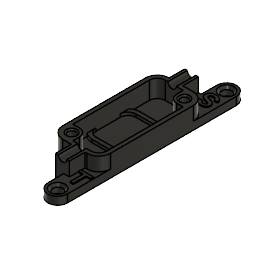
PE3 - PCB Case (Autodesk Fusion 360 design; units mm, degrees)
Autodesk Fusion 360 part; units mm, degrees
sketch "Sketch1" plane through (0, 0, 0) normal (0, 0, 1) x (1, 0, 0)
  line L0 (6.2013, 10.25) -> (-6.2012, 10.25)
  line L1 (-10.25, 6.2013) -> (-10.25, -6.2012)
  line L2 (-6.2012, -10.25) -> (6.2013, -10.25)
  line L3 (10.25, -6.2012) -> (10.25, 6.2012)
  line L4 (10.25, 10.25) -> (-10.25, -10.25) construction
  line L5 (-10.25, 10.25) -> (10.25, -10.25) construction
  arc A0 (-6.2012, 10.25) -> (-10.25, 6.2013) centre (-6.2013, 6.2013) ccw
  arc A1 (10.25, 6.2012) -> (6.2013, 10.25) centre (6.2012, 6.2012) ccw
  arc A2 (-10.25, -6.2012) -> (-6.2012, -10.25) centre (-6.2013, -6.2013) ccw
  arc A3 (6.2013, -10.25) -> (10.25, -6.2012) centre (6.2013, -6.2013) ccw
  line L6 (-12.25, 6.2013) -> (-12.25, -6.2013)
  arc A4 (-12.25, -6.2012) -> (-6.2012, -12.25) centre (-6.2013, -6.2013) ccw
  line L7 (-6.2012, -12.25) -> (6.2013, -12.25)
  arc A5 (6.2013, -12.25) -> (12.25, -6.2012) centre (6.2013, -6.2013) ccw
  line L8 (12.25, -6.2012) -> (12.25, 6.2012)
  arc A6 (12.25, 6.2012) -> (6.2013, 12.25) centre (6.2012, 6.2012) ccw
  line L9 (6.2013, 12.25) -> (-6.2012, 12.25)
  arc A7 (-6.2012, 12.25) -> (-12.25, 6.2013) centre (-6.2013, 6.2013) ccw
  dimension "d1" = 20.5
  dimension "d2" = 20.5
  dimension "d3" = 4.0488
  dimension "d4" = 4.0488
  dimension "d5" = 4.0488
  dimension "d6" = 4.0488
  dimension "d7" = 2
  constraint horizontal L0
  constraint perpendicular L0 L1
  constraint parallel L0 L2
  constraint parallel L1 L3
  constraint coincident L4 origin
  constraint coincident L5 origin
  constraint coincident L5.start L0
  constraint coincident L5.start L1
  constraint tangent L0 A0
  constraint tangent L1 A0
  constraint coincident L4.start L0
  constraint coincident L4.start L3
  constraint tangent L0 A1
  constraint tangent L3 A1
  constraint coincident L4.end L2
  constraint coincident L4.end L1
  constraint tangent L2 A2
  constraint tangent L1 A2
  constraint coincident L5.end L3
  constraint coincident L5.end L2
  constraint tangent L3 A3
  constraint tangent L2 A3
  measures "d1" distance of L4.start L5.start
  measures "d2" distance of L4.start L5.end
  measures "d3" radius of A0
  measures "d4" radius of A1
  measures "d5" radius of A2
  measures "d6" radius of A3
extrude "Extrude1" add sketch "Sketch1" along normal blind 6 contours L0 L1 L2 L3 A0 A1 A2 A3 | L6 A4 L7 A5 L8 A6 L9 A7
extrude "Extrude2" add sketch "Sketch1" along normal blind 1.5 from surface at 6
sketch "Sketch10" plane through (0, 0, 0) normal (0, 0, 1) x (1, 0, 0)
  line L0 (7.2501, -43.2789) -> (7.2501, 43.2211) construction
  line L1 (7.2501, -0.0289) -> (8.1135, -0.0289) construction
  circle A0 centre (7.2501, 43.2211) radius 2.5
  circle A1 centre (7.2501, -43.2789) radius 2.5
  arc A2 (2.2502, -43.2493) -> (12.25, -43.25) centre (7.2501, -43.2789) ccw
  arc A3 (12.25, 43.1922) -> (2.2502, 43.1914) centre (7.2501, 43.2211) ccw
  line L2 (2.2502, 43.1914) -> (2.2502, -43.3086)
  line L3 (12.25, -43.25) -> (12.25, 43.25)
  dimension "d42" = 86.5
  dimension "d43" = 5
  dimension "d44" = 5
  dimension "d45" = 10
  dimension "d46" = 10
  dimension "d134" = 0.0289
  dimension "d135" = 7.2501
  dimension "d136" = 0.8634
  constraint midpoint L0 L1.start
  constraint perpendicular L0 L1
  constraint coincident L0.end A0.centre
  constraint coincident L0.start A1.centre
  constraint concentric A1 A2
  constraint concentric A0 A3
  constraint parallel L0 L2
  constraint coincident A2 L2.end
  constraint coincident L2 A2.start
  constraint vertical L3
  constraint coincident L3 A3.start
  constraint coincident A3 L3.end
  constraint parallel L0 L3
  constraint equal L0 L2
  constraint equal L0 L3
  measures "d42" distance of L0.start L0.end
  measures "d43" diameter of A0
  measures "d44" diameter of A1
  measures "d45" diameter of A2
  measures "d46" diameter of A3
  measures "d134" distance of origin L1
  measures "d135" distance of origin L0
  measures "d136" distance of L0 L1.end
extrude "Extrude10" add sketch "Sketch10" along normal blind 4
chamfer "Chamfer1" distance 1.25 angle 45 2 edges at (6.346, -45.6097, 4) (6.346, 40.8903, 4)
sketch "Sketch12" plane through (0, 0, 0) normal (0, 0, -1) x (1, 0, 0)
  circle A0 centre (7.2501, 43.2789) radius 2.5
  circle A1 centre (7.2501, -43.2211) radius 2.5
  line L0 (2.2502, 12.25) -> (-6.2012, 12.25)
  arc A2 (-6.2013, 12.25) -> (-12.25, 6.2012) centre (-6.2013, 6.2013) ccw
  line L1 (-12.25, 6.2012) -> (-12.25, -6.2013)
  arc A3 (-12.25, -6.2013) -> (-6.2012, -12.25) centre (-6.2013, -6.2013) ccw
  line L2 (2.2502, -12.25) -> (2.2502, -43.1914)
  arc A4 (2.2502, -43.1914) -> (12.25, -43.25) centre (7.2501, -43.2211) ccw
  line L3 (12.25, -43.25) -> (12.25, 43.25)
  arc A5 (12.25, 43.25) -> (2.2502, 43.3086) centre (7.2501, 43.2789) ccw
  line L4 (10.25, -21.2012) -> (10.25, 21.2013)
  arc A6 (-6.2013, 25.25) -> (-10.25, 21.2013) centre (-6.2013, 21.2013) ccw
  arc A7 (-12.25, -21.2012) -> (-6.2013, -27.25) centre (-6.2013, -21.2012) ccw
  arc A8 (6.2013, -25.25) -> (10.25, -21.2012) centre (6.2013, -21.2012) ccw
  line L5 (-10.25, 25.25) -> (10.25, -25.25) construction
  line L6 (10.25, 25.25) -> (-10.25, -25.25) construction
  line L7 (-12.25, 21.2012) -> (-12.25, -21.2012)
  line L8 (-10.25, 21.2013) -> (-10.25, -21.2012)
  arc A9 (12.25, 21.2013) -> (6.2013, 27.25) centre (6.2012, 21.2013) ccw
  arc A10 (-6.2012, 27.25) -> (-12.25, 21.2012) centre (-6.2013, 21.2013) ccw
  line L9 (-6.2013, -25.25) -> (6.2013, -25.25)
  line L10 (6.2012, 25.25) -> (-6.2013, 25.25)
  line L11 (12.25, -21.2012) -> (12.25, 21.2013)
  arc A11 (10.25, 21.2013) -> (6.2012, 25.25) centre (6.2012, 21.2013) ccw
  arc A12 (-10.25, -21.2012) -> (-6.2013, -25.25) centre (-6.2013, -21.2012) ccw
  arc A13 (6.2012, -27.25) -> (12.25, -21.2012) centre (6.2013, -21.2012) ccw
  line L12 (-6.2013, -27.25) -> (6.2012, -27.25)
  line L13 (6.2013, 27.25) -> (-6.2012, 27.25)
  line L14 (-6.2012, -12.25) -> (2.2502, -12.25)
  line L15 (2.2502, 43.3086) -> (2.2502, 12.25)
  dimension "d77" = 2
  dimension "d78" = 20.5
  dimension "d79" = 50.5
  dimension "d80" = 4.0488
  dimension "d81" = 4.0488
  dimension "d82" = 4.0488
  dimension "d83" = 4.0488
  constraint horizontal L10
  constraint perpendicular L8 L10
  constraint parallel L9 L10
  constraint parallel L4 L8
  constraint coincident origin L6
  constraint coincident origin L5
  constraint coincident L5.start L10
  constraint coincident L5.start L8
  constraint tangent A6 L10
  constraint tangent A6 L8
  constraint coincident L6.start L10
  constraint coincident L6.start L4
  constraint tangent L10 A11
  constraint tangent L4 A11
  constraint coincident L6.end L9
  constraint coincident L6.end L8
  constraint tangent L9 A12
  constraint tangent L8 A12
  constraint coincident L5.end L4
  constraint coincident L5.end L9
  constraint tangent L4 A8
  constraint tangent A8 L9
  measures "d78" distance of L5.start L6.start
  measures "d79" distance of L5.end L6.start
  measures "d80" radius of A6
  measures "d81" radius of A11
  measures "d82" radius of A12
  measures "d83" radius of A8
extrude "Extrude13" cut 1 faces at (-3.4167, 2.0671, 6) along direction (0, 0, -1) blind 1
extrude "Extrude14" add sketch "Sketch12" against normal blind 11 contours L2 L3 L4 A8 A9 L9 L10 L11 A11 A13 L12 L13 L15 | A2 A6 L7 L8 A10 L10 L13 L15 | A2 L1 A3 L7 L8 | A3 L2 A7 L7 L8 L9 A12 L12
extrude "Extrude15" add sketch "Sketch12" against normal blind 4 contours L0 A2 A6 L8 L10 L15 | A3 L2 L8 L9 A12 L14
sketch "Sketch13" plane through (0, -27.25, 0) normal (0, -1, 0) x (1, 0, 0)
  line L0 (2.2502, 0) -> (2.2502, 4)
  line L1 (2.2502, 4) -> (6.2013, 4)
  line L2 (6.2013, 4) -> (6.2013, 11)
  line L3 (6.2013, 11) -> (-6.2012, 11)
  line L4 (-6.2012, 11) -> (-6.2012, 0)
  line L5 (-6.2012, 0) -> (2.2502, 0)
  line L6 (-1.8, 0) -> (5.2012, 0)
  line L7 (5.2012, 11) -> (5.2012, 0)
  line L8 (6.2012, 4) -> (3.0821, 4)
  line L9 (-1.8, 11) -> (-1.8, -1.0165)
  line L10 (-1.8, 0) -> (5.2012, 0)
  line L11 (-1.8, -1.0165) -> (-1.8, 0)
  line L12 (3.85, 11) -> (5.2012, 11)
  line L13 (-0.45, 11) -> (-1.8, 11)
  arc A0 (-0.45, 11) -> (3.85, 11) centre (1.7, 11) ccw
  point P0 (1.7, 11)
  dimension "d89" = 7
  dimension "d90" = 4.3
  constraint horizontal L10
  constraint horizontal L8
  constraint coincident P0 A0.centre
  constraint coincident L6.end L7.end
  constraint perpendicular L6 L7
  constraint perpendicular L10 L11
  constraint coincident L5 L6.start
  constraint perpendicular L7 L12
  constraint perpendicular L9 L13
  measures "d89" distance of L9.end L8.end
  measures "d90" diameter of A0
sketch "Sketch14" plane through (0, 27.25, 0) normal (0, 1, 0) x (-1, 0, 0)
  line L0 (-2.2502, 4) -> (-2.2502, 0)
  line L1 (-2.2502, 0) -> (6.2013, 0)
  line L2 (6.2013, 0) -> (6.2013, 11)
  line L3 (6.2013, 11) -> (-6.2012, 11)
  line L4 (-6.2012, 11) -> (-6.2012, 4)
  line L5 (-6.2012, 4) -> (-2.2502, 4)
  line L6 (-6.2013, 0) -> (-6.2013, 4)
  line L7 (-0.8, 15) -> (-0.8, 4)
  line L8 (-6.2013, 0) -> (6.2012, 0)
  line L9 (-0.8, 15) -> (6.2012, 15)
  line L10 (6.2012, 4) -> (6.2, 4)
  line L11 (6.2012, 15) -> (6.2012, 0)
  circle A0 centre (2.7, 11) radius 2.15
  line L12 (-0.8, 4) -> (-6.2013, 4)
  line L13 (-6.2013, 0) -> (6.2012, 0)
  point P0 (2.7, 11)
  dimension "d91" = 7
  dimension "d92" = 4.3
  dimension "d137" = 12.4012
  dimension "d138" = 7
  dimension "d139" = 11
  dimension "d140" = 0.0012
  dimension "d141" = 3.5
  constraint horizontal L13
  constraint horizontal L10
  constraint collinear L10 L12
  constraint coincident P0 A0.centre
  constraint coincident L8.end L11.end
  constraint perpendicular L8 L11
  constraint coincident L6.start L8.start
  constraint perpendicular L6 L12
  constraint coincident L4.end L6.end
  constraint perpendicular L7 L12
  constraint equal L0 L6
  constraint coincident L10.start L11
  constraint perpendicular L7 L9
  constraint coincident L1 origin
  measures "d91" distance of L7.end L10.end
  measures "d92" diameter of A0
  measures "d137" distance of L4 L10.end
  measures "d138" distance of L5 P0
  measures "d139" distance of L10.start L9
  measures "d140" distance of L10.end L11
  measures "d141" distance of P0 L7
extrude "Extrude16" add sketch "Sketch13" along normal blind 8 contours L0 L1 L3 L5 L6 L7 L8 L9 L10 L12 L13 A0
extrude "Extrude17" add sketch "Sketch13" along normal blind 8 contours L0 L1 L3 L5 L6 L7 L8 L9 L10 L12 L13 A0
extrude "Extrude18" add sketch "Sketch14" along normal blind 8 contours L0 L1 L2 L3 L7 L8 L11 A0 L12 L13
extrude "Extrude19" cut 1 faces at (-2.4382, 27.25, 10.3329) along direction (0, -1, 0) blind 5
extrude "Extrude20" cut 1 faces at (1.4382, -27.25, 10.3329) along direction (0, 1, 0) blind 4
sketch "Sketch15" plane through (0, 0, 4) normal (0, 0, 1) x (-1, 0, 0)
  line L0 (-10.25, 21.2013) -> (-10.25, 10.6951)
  arc A0 (-6.2013, 12.25) -> (-10.25, 10.6951) centre (-6.2013, 6.2013) ccw
  line L1 (-6.2013, 12.25) -> (6.2013, 12.25)
  arc A1 (10.25, 10.6951) -> (6.2012, 12.25) centre (6.2013, 6.2013) ccw
  line L2 (10.25, 10.6951) -> (10.25, 21.2013)
  arc A2 (10.25, 21.2013) -> (6.2013, 25.25) centre (6.2013, 21.2013) ccw
  line L3 (6.2013, 25.25) -> (-6.2012, 25.25)
  arc A3 (-6.2012, 25.25) -> (-10.25, 21.2013) centre (-6.2012, 21.2013) ccw
  circle A4 centre (6.9428, 21.9428) radius 2
  line L4 (8.8794, 25.9428) -> (2.9428, 25.9428)
  line L5 (2.9428, 25.9428) -> (2.9428, 21.9428)
  line L6 (6.9428, 17.9428) -> (10.9428, 17.9428)
  line L7 (10.9428, 17.9428) -> (10.9428, 23.8794)
  arc A5 (2.9428, 21.9428) -> (6.9428, 17.9428) centre (6.9428, 21.9428) ccw
  line L8 (10.9428, 17.9428) -> (10.9428, 23.8794)
  line L9 (8.8794, 25.9428) -> (2.9428, 25.9428)
  line L10 (2.9428, 25.9428) -> (2.9428, 21.9428)
  line L11 (6.9428, 17.9428) -> (10.9428, 17.9428)
  arc A6 (2.9428, 21.9428) -> (6.9428, 17.9428) centre (6.9428, 21.9428) ccw
  circle A7 centre (6.9428, 21.9428) radius 2
  line L12 (-1.75, 0) -> (-22.5, 0) construction
  line L13 (0, -2.5) -> (0, -20) construction
  line L14 (-8.0247, -25.9428) -> (-2.9428, -25.9428)
  line L15 (-2.9428, -25.9428) -> (-2.9428, -21.9428)
  arc A8 (-2.9428, -21.9428) -> (-6.9428, -17.9428) centre (-6.9428, -21.9428) ccw
  line L16 (-10.9428, -17.9428) -> (-10.9428, -23.0247)
  line L17 (-6.9428, -17.9428) -> (-10.9428, -17.9428)
  circle A9 centre (-6.9428, -21.9428) radius 2
  line L18 (-8.0247, -25.9428) -> (-10.9428, -23.0247)
  line L19 (-8.0247, -25.9428) -> (-3.8978, -25.9428) construction
  line L20 (10.9428, 23.8794) -> (8.8794, 25.9428)
  point P0 (6.9428, 21.9428)
  dimension "d106" = 4
  dimension "d109" = 4
  dimension "d114" = 4
  dimension "d115" = 4
  dimension "d116" = 135
  dimension "d142" = 17.9428
  dimension "d143" = 25.9428
  dimension "d144" = 23.0247
  dimension "d145" = 5.8857
  dimension "d149" = 23.8794
  dimension "d150" = 5.9366
  dimension "d151" = 17.9428
  dimension "d152" = 8
  constraint horizontal L4
  constraint perpendicular L4 L5
  constraint parallel L4 L6
  constraint parallel L5 L7
  constraint tangent L5 A5
  constraint tangent L6 A5
  constraint horizontal L9
  constraint perpendicular L9 L10
  constraint parallel L9 L11
  constraint parallel L8 L10
  constraint tangent L10 A6
  constraint tangent L11 A6
  constraint horizontal L19
  constraint tangent A8 L17
  constraint tangent L15 A8
  constraint concentric A8 A9
  constraint concentric A5 A7
  constraint equal A5 A8
  constraint midpoint A5 A6
  constraint equal L5 L10
  constraint equal L5 L11
  constraint equal L5 L15
  constraint equal L5 L17
  constraint perpendicular L16 L17
  constraint equal L18 L19
  constraint equal A4 A9
  constraint concentric A4 A5
  constraint coincident P0 A4.centre
  measures "d106" diameter of A4
  measures "d109" radius of A5
  measures "d114" diameter of A7
  measures "d115" radius of A6
  measures "d116" angle of L18 L19
  measures "d142" distance of L12 L17
  measures "d143" distance of L12 L19
  measures "d144" distance of L12 L16.end
  measures "d145" distance of L5 L15
  measures "d149" distance of L12 L7.end
  measures "d150" distance of L5 L4.start
  measures "d151" distance of L6 L12
  measures "d152" distance of L5 L7
extrude "Extrude21" add sketch "Sketch15" along normal blind 7 contours L2 A2 L3 L5 L6 A5 L10 L11 A6 | L14 L15 A8 L16 L17 L18
chamfer "Chamfer5" distance 0.7 angle 45 2 edges at (8.8075, 21.2196, 11) (-5.0782, -22.6661, 11)
extrude "Extrude24" cut 2 faces at (3.0992, -19.4386, 4) (-3.0992, 19.4386, 4) along direction (0, 0, -1) blind 2
extrude "Extrude25" cut 1 faces at (-3.4167, 2.0671, 5) along direction (0, 0, -1) blind 3
sketch "Sketch16" plane through (0, 0, 4) normal (0, 0, 1) x (-1, 0, 0)
  arc A0 (-12.25, -21.2012) -> (-6.2012, -27.25) centre (-6.2013, -21.2012) ccw
  line L0 (-12.25, -21.2012) -> (-12.25, -43.25)
  arc A1 (-12.25, -43.25) -> (-2.2502, -43.1914) centre (-7.2501, -43.2211) ccw
  line L1 (-2.2502, -43.1914) -> (-2.2502, -35.25)
  line L2 (-2.2502, -35.25) -> (-0.8, -35.25)
  line L3 (-0.8, -35.25) -> (-0.8, -27.25)
  line L4 (-10.7579, -32.3932) -> (-6.9514, -32.3932) construction
  line L5 (-6.9514, -32.3932) -> (-6.9514, -27.9161) construction
  line L6 (-6.9514, -27.9161) -> (-10.7579, -27.9161) construction
  line L7 (-10.7579, -27.9161) -> (-10.7579, -32.3932) construction
  line L8 (-0.8, -27.25) -> (-6.2012, -27.25)
  circle A2 centre (-7.2501, -43.2211) radius 3.75
  dimension "d124" = 8
  dimension "d153" = 5.2986
  dimension "d154" = 15.3339
  dimension "d155" = 3.8065
  dimension "d156" = 4.4771
  text T0 "S" font "Arial" height 8 bold align left top in box 3.8065 x 4.4771 at (-10.7579, -32.3932) x (1, 0) y (0, 1) spacing 1 kerned
  measures "d153" distance of L0 L5
  measures "d154" distance of L0.end L6
  measures "d155" distance of L5 L7
  measures "d156" distance of L4 L6
extrude "Extrude26" add sketch "Sketch16" along normal blind 0.5 text T0
sketch "Sketch17" plane through (0, 0, 4) normal (0, 0, 1) x (-1, 0, 0)
  circle A0 centre (-7.2501, 43.2789) radius 3.75
  line L0 (-5.2012, 27.25) -> (-5.2012, 35.25)
  line L1 (-5.2012, 35.25) -> (-2.2502, 35.25)
  line L2 (-2.2502, 35.25) -> (-2.2502, 43.3086)
  arc A1 (-2.2502, 43.3086) -> (-12.25, 43.25) centre (-7.2501, 43.2789) ccw
  line L3 (-12.25, 43.25) -> (-12.25, 21.2013)
  arc A2 (-6.2013, 27.25) -> (-12.25, 21.2013) centre (-6.2012, 21.2013) ccw
  line L4 (-6.2013, 27.25) -> (-5.2012, 27.25)
  line L5 (-5.3111, 31.9604) -> (-9.1175, 31.9604) construction
  line L6 (-9.1175, 31.9604) -> (-9.1175, 27.4833) construction
  line L7 (-9.1175, 27.4833) -> (-5.3111, 27.4833) construction
  line L8 (-5.3111, 27.4833) -> (-5.3111, 31.9604) construction
  dimension "d127" = 8
  dimension "d157" = 6.9389
  dimension "d158" = 6.282
  dimension "d159" = 4.4771
  dimension "d160" = 3.8065
  text T0 "T" font "Arial" height 8 bold align left top in box 3.8065 x 4.4771 at (-5.3111, 31.9604) x (-1, 0) y (0, -1) spacing 1 kerned
  constraint vertical L8
  measures "d157" distance of L3 L8
  measures "d158" distance of L3.end L7
  measures "d159" distance of L5 L7
  measures "d160" distance of L6 L8
extrude "Extrude27" add sketch "Sketch17" along normal blind 0.5 text T0
extrude "Extrude28" cut 2 faces at (-2.0671, 10.9167, 7.5) (-2.0671, -11.5833, 7.5) along direction (0, 0, -1) blind 4
equation "d3 = ( 20.5 / 20 * 3.95 ) * 1 mm"
equation "d4 = ( 20.5 / 20 * 3.95 ) * 1 mm"
equation "d5 = ( 20.5 / 20 * 3.95 ) * 1 mm"
equation "d6 = ( 20.5 / 20 * 3.95 ) * 1 mm"
equation "d80 = ( 20.5 / 20 * 3.95 ) * 1 mm"
equation "d81 = ( 20.5 / 20 * 3.95 ) * 1 mm"
equation "d82 = ( 20.5 / 20 * 3.95 ) * 1 mm"
equation "d83 = ( 20.5 / 20 * 3.95 ) * 1 mm"
